Autodesk Inventor part; units mm, degrees
(part 2 of 2)
  spline S171 degree 2 poles (10.8818, -199.8751) (10.7521, -199.927) (10.5113, -200.0752) (10.4372, -200.1271) knots 0 0 0 1 2 2 2
  line L143 (10.4372, -200.1271) -> (10.4038, -200.1271)
  line L144 (10.4038, -200.1271) -> (10.4038, -199.475)
  spline S172 degree 2 poles (10.4038, -199.475) (10.5928, -199.3824) (11.2708, -199.2008) (11.5746, -199.2008) knots 0 0 0 1 2 2 2
  spline S173 degree 2 poles (11.5746, -199.2008) (12.2156, -199.2008) (12.938, -199.8788) (12.938, -200.4568) knots 0 0 0 1 2 2 2
  spline S174 degree 2 poles (12.938, -200.4568) (12.938, -200.7273) (12.8121, -201.1793) (12.7009, -201.372) knots 0 0 0 1 2 2 2
  spline S175 degree 2 poles (12.7009, -201.372) (12.5898, -201.572) (12.2674, -201.9648) (12.0896, -202.1537) knots 0 0 0 1 2 2 2
  spline S176 degree 2 poles (12.0896, -202.1537) (11.8006, -202.4686) (11.0929, -203.143) (10.8818, -203.3393) knots 0 0 0 1 2 2 2
  line L145 (10.8818, -203.3393) -> (13.127, -203.3393)
  line L146 (13.127, -203.3393) -> (13.127, -203.8691)
  line L147 (16.6801, -202.2982) -> (16.1355, -202.2982)
  line L148 (16.1355, -202.2982) -> (16.1355, -203.8691)
  line L149 (16.1355, -203.8691) -> (15.5464, -203.8691)
  line L150 (15.5464, -203.8691) -> (15.5464, -202.2982)
  line L151 (15.5464, -202.2982) -> (13.5271, -202.2982)
  line L152 (13.5271, -202.2982) -> (13.5271, -201.6535)
  line L153 (13.5271, -201.6535) -> (15.5723, -199.2971)
  line L154 (15.5723, -199.2971) -> (16.1355, -199.2971)
  line L155 (16.1355, -199.2971) -> (16.1355, -201.8054)
  line L156 (16.1355, -201.8054) -> (16.6801, -201.8054)
  line L157 (16.6801, -201.8054) -> (16.6801, -202.2982)
  line L158 (15.5464, -201.8054) -> (15.5464, -200.0196)
  line L159 (15.5464, -200.0196) -> (14.0088, -201.8054)
  line L160 (14.0088, -201.8054) -> (15.5464, -201.8054)
  line L161 (19.0699, -199.0934) -> (17.2803, -204.8621)
  line L162 (17.2803, -204.8621) -> (16.7616, -204.8621)
  line L163 (16.7616, -204.8621) -> (18.5437, -199.0934)
  line L164 (18.5437, -199.0934) -> (19.0699, -199.0934)
  line L165 (22.3933, -203.8691) -> (19.5737, -203.8691)
  line L166 (19.5737, -203.8691) -> (19.5737, -203.2208)
  spline S177 degree 2 poles (19.5737, -203.2208) (19.8776, -202.9355) (20.4185, -202.4057) (20.6778, -202.1204) knots 0 0 0 1 2 2 2
  spline S178 degree 2 poles (20.6778, -202.1204) (21.2003, -201.5461) (21.5819, -200.857) (21.5819, -200.4902) knots 0 0 0 1 2 2 2
  spline S179 degree 2 poles (21.5819, -200.4902) (21.5819, -200.2975) (21.4633, -200.0085) (21.3559, -199.9159) knots 0 0 0 1 2 2 2
  spline S180 degree 2 poles (21.3559, -199.9159) (21.2484, -199.8233) (20.9668, -199.7306) (20.7964, -199.7306) knots 0 0 0 1 2 2 2
  spline S181 degree 2 poles (20.7964, -199.7306) (20.6334, -199.7306) (20.2999, -199.8121) (20.148, -199.8751) knots 0 0 0 1 2 2 2
  spline S182 degree 2 poles (20.148, -199.8751) (20.0183, -199.927) (19.7775, -200.0752) (19.7034, -200.1271) knots 0 0 0 1 2 2 2
  line L167 (19.7034, -200.1271) -> (19.6701, -200.1271)
  line L168 (19.6701, -200.1271) -> (19.6701, -199.475)
  spline S183 degree 2 poles (19.6701, -199.475) (19.859, -199.3824) (20.5371, -199.2008) (20.8409, -199.2008) knots 0 0 0 1 2 2 2
  spline S184 degree 2 poles (20.8409, -199.2008) (21.4818, -199.2008) (22.2043, -199.8788) (22.2043, -200.4568) knots 0 0 0 1 2 2 2
  spline S185 degree 2 poles (22.2043, -200.4568) (22.2043, -200.7273) (22.0783, -201.1793) (21.9672, -201.372) knots 0 0 0 1 2 2 2
  spline S186 degree 2 poles (21.9672, -201.372) (21.856, -201.572) (21.5337, -201.9648) (21.3559, -202.1537) knots 0 0 0 1 2 2 2
  spline S187 degree 2 poles (21.3559, -202.1537) (21.0669, -202.4686) (20.3592, -203.143) (20.148, -203.3393) knots 0 0 0 1 2 2 2
  line L169 (20.148, -203.3393) -> (22.3933, -203.3393)
  line L170 (22.3933, -203.3393) -> (22.3933, -203.8691)
  spline S188 degree 2 poles (25.8501, -201.5831) (25.8501, -202.8132) (25.135, -203.9655) (24.3903, -203.9655) knots 0 0 0 1 2 2 2
  spline S189 degree 2 poles (24.3903, -203.9655) (23.6345, -203.9655) (22.9268, -202.791) (22.9268, -201.5868) knots 0 0 0 1 2 2 2
  spline S190 degree 2 poles (22.9268, -201.5868) (22.9268, -200.3494) (23.6419, -199.2045) (24.3903, -199.2045) knots 0 0 0 1 2 2 2
  spline S191 degree 2 poles (24.3903, -199.2045) (25.1424, -199.2045) (25.8501, -200.3901) (25.8501, -201.5831) knots 0 0 0 1 2 2 2
  spline S192 degree 2 poles (25.0646, -202.9762) (25.1535, -202.7502) (25.2276, -202.0537) (25.2276, -201.5831) knots 0 0 0 1 2 2 2
  spline S193 degree 2 poles (25.2276, -201.5831) (25.2276, -201.1126) (25.1535, -200.4198) (25.0609, -200.1863) knots 0 0 0 1 2 2 2
  spline S194 degree 2 poles (25.0609, -200.1863) (24.9683, -199.9529) (24.6459, -199.7121) (24.3903, -199.7121) knots 0 0 0 1 2 2 2
  spline S195 degree 2 poles (24.3903, -199.7121) (24.1346, -199.7121) (23.8049, -199.9529) (23.7086, -200.1938) knots 0 0 0 1 2 2 2
  spline S196 degree 2 poles (23.7086, -200.1938) (23.6159, -200.4272) (23.5492, -201.1385) (23.5492, -201.5868) knots 0 0 0 1 2 2 2
  spline S197 degree 2 poles (23.5492, -201.5868) (23.5492, -202.0685) (23.6085, -202.7132) (23.7048, -202.9651) knots 0 0 0 1 2 2 2
  spline S198 degree 2 poles (23.7048, -202.9651) (23.7938, -203.2022) (24.1235, -203.4579) (24.3903, -203.4579) knots 0 0 0 1 2 2 2
  spline S199 degree 2 poles (24.3903, -203.4579) (24.6422, -203.4579) (24.972, -203.2171) (25.0646, -202.9762) knots 0 0 0 1 2 2 2
  line L171 (29.255, -203.8691) -> (26.4355, -203.8691)
  line L172 (26.4355, -203.8691) -> (26.4355, -203.2208)
  spline S200 degree 2 poles (26.4355, -203.2208) (26.7393, -202.9355) (27.2802, -202.4057) (27.5395, -202.1204) knots 0 0 0 1 2 2 2
  spline S201 degree 2 poles (27.5395, -202.1204) (28.062, -201.5461) (28.4436, -200.857) (28.4436, -200.4902) knots 0 0 0 1 2 2 2
  spline S202 degree 2 poles (28.4436, -200.4902) (28.4436, -200.2975) (28.325, -200.0085) (28.2176, -199.9159) knots 0 0 0 1 2 2 2
  spline S203 degree 2 poles (28.2176, -199.9159) (28.1101, -199.8233) (27.8285, -199.7306) (27.6581, -199.7306) knots 0 0 0 1 2 2 2
  spline S204 degree 2 poles (27.6581, -199.7306) (27.4951, -199.7306) (27.1616, -199.8121) (27.0097, -199.8751) knots 0 0 0 1 2 2 2
  spline S205 degree 2 poles (27.0097, -199.8751) (26.8801, -199.927) (26.6392, -200.0752) (26.5651, -200.1271) knots 0 0 0 1 2 2 2
  line L173 (26.5651, -200.1271) -> (26.5318, -200.1271)
  line L174 (26.5318, -200.1271) -> (26.5318, -199.475)
  spline S206 degree 2 poles (26.5318, -199.475) (26.7207, -199.3824) (27.3988, -199.2008) (27.7026, -199.2008) knots 0 0 0 1 2 2 2
  spline S207 degree 2 poles (27.7026, -199.2008) (28.3435, -199.2008) (29.066, -199.8788) (29.066, -200.4568) knots 0 0 0 1 2 2 2
  spline S208 degree 2 poles (29.066, -200.4568) (29.066, -200.7273) (28.94, -201.1793) (28.8289, -201.372) knots 0 0 0 1 2 2 2
  spline S209 degree 2 poles (28.8289, -201.372) (28.7177, -201.572) (28.3954, -201.9648) (28.2176, -202.1537) knots 0 0 0 1 2 2 2
  spline S210 degree 2 poles (28.2176, -202.1537) (27.9286, -202.4686) (27.2209, -203.143) (27.0097, -203.3393) knots 0 0 0 1 2 2 2
  line L175 (27.0097, -203.3393) -> (29.255, -203.3393)
  line L176 (29.255, -203.3393) -> (29.255, -203.8691)
  spline S211 degree 2 poles (32.7562, -202.3871) (32.7562, -202.7391) (32.5228, -203.3356) (32.3264, -203.5357) knots 0 0 0 1 2 2 2
  spline S212 degree 2 poles (32.3264, -203.5357) (32.1227, -203.7469) (31.6114, -203.9655) (31.3039, -203.9655) knots 0 0 0 1 2 2 2
  spline S213 degree 2 poles (31.3039, -203.9655) (30.9963, -203.9655) (30.4887, -203.758) (30.2961, -203.5505) knots 0 0 0 1 2 2 2
  spline S214 degree 2 poles (30.2961, -203.5505) (30.059, -203.3023) (29.7922, -202.4686) (29.7922, -201.861) knots 0 0 0 1 2 2 2
  spline S215 degree 2 poles (29.7922, -201.861) (29.7922, -201.2645) (30.0367, -200.3049) (30.2924, -199.9492) knots 0 0 0 1 2 2 2
  spline S216 degree 2 poles (30.2924, -199.9492) (30.5406, -199.601) (31.3261, -199.2119) (31.8411, -199.2119) knots 0 0 0 1 2 2 2
  spline S217 degree 2 poles (31.8411, -199.2119) (31.993, -199.2119) (32.2597, -199.2416) (32.3598, -199.2749) knots 0 0 0 1 2 2 2
  line L177 (32.3598, -199.2749) -> (32.3598, -199.864)
  line L178 (32.3598, -199.864) -> (32.3338, -199.864)
  spline S218 degree 2 poles (32.3338, -199.864) (32.2486, -199.8196) (31.9374, -199.7417) (31.7596, -199.7417) knots 0 0 0 1 2 2 2
  spline S219 degree 2 poles (31.7596, -199.7417) (31.189, -199.7417) (30.4887, -200.5124) (30.4221, -201.2682) knots 0 0 0 1 2 2 2
  spline S220 degree 2 poles (30.4221, -201.2682) (30.6407, -201.1163) (31.1001, -200.9496) (31.3742, -200.9496) knots 0 0 0 1 2 2 2
  spline S221 degree 2 poles (31.3742, -200.9496) (31.641, -200.9496) (32.0412, -201.057) (32.2597, -201.22) knots 0 0 0 1 2 2 2
  spline S222 degree 2 poles (32.2597, -201.22) (32.5117, -201.409) (32.7562, -201.9944) (32.7562, -202.3871) knots 0 0 0 1 2 2 2
  spline S223 degree 2 poles (32.1338, -202.4131) (32.1338, -202.1315) (31.9856, -201.7499) (31.8226, -201.6165) knots 0 0 0 1 2 2 2
  spline S224 degree 2 poles (31.8226, -201.6165) (31.7003, -201.5202) (31.3965, -201.4572) (31.2372, -201.4572) knots 0 0 0 1 2 2 2
  spline S225 degree 2 poles (31.2372, -201.4572) (31.0223, -201.4572) (30.6184, -201.5868) (30.4221, -201.7091) knots 0 0 0 1 2 2 2
  spline S226 degree 2 poles (30.4221, -201.7091) (30.4184, -201.7758) (30.4109, -201.9018) (30.4109, -201.9981) knots 0 0 0 1 2 2 2
  spline S227 degree 2 poles (30.4109, -201.9981) (30.4109, -202.4723) (30.5962, -203.054) (30.737, -203.2059) knots 0 0 0 1 2 2 2
  spline S228 degree 2 poles (30.737, -203.2059) (30.8667, -203.3504) (31.1482, -203.4653) (31.3076, -203.4653) knots 0 0 0 1 2 2 2
  spline S229 degree 2 poles (31.3076, -203.4653) (31.6781, -203.4653) (32.1338, -202.9392) (32.1338, -202.4131) knots 0 0 0 1 2 2 2
  point P0 (0, 0)
  constraints: 2 other
emboss "Emboss1" sketch "Sketch14" operation cut depth 2.54 direction (-1, 0, 0)
sketch "Sketch16" plane through (5.08, 0, 0) normal (1, 0, 0) x (0, 0, -1)
  line L0 (-45.5467, -73.9362) -> (38.2733, -73.9362)
  line L1 (38.2733, -73.9362) -> (38.2733, -77.7462)
  line L2 (38.2733, -77.7462) -> (-45.5467, -77.7462)
  line L3 (-45.5467, -77.7462) -> (-45.5467, -73.9362)
  line L4 (38.9083, -211.0962) -> (-46.1817, -211.0962) projected
  line L5 (42.0833, 28.0448) -> (42.0833, -207.9212) projected
  line L6 (-49.3567, -207.9212) -> (-49.3567, 28.0448) projected
  point P0 (0, 0)
  point P1 (38.9083, -223.7962)
  point P2 (42.0833, -220.6212)
  point P3 (38.2733, -75.8412)
  point P4 (-45.5467, -75.8412)
  dimension "d195" = 3.81
  dimension "d692" = 137.16
  dimension "d796" = 3.81
  dimension "d797" = 3.81
  constraints: 8 end point, 2 midpoint, 2 parallel, 1 horizontal, 1 perpendicular, 1 other
  measures "d195" distance between parallel lines of L0 L2
  measures "d796" distance from line of L5 point (38.273, -75.841)
  measures "d797" distance from line of L6 point (-45.547, -75.841)
extrude "Extrusion13" add sketch "Sketch16" along normal blind 5.08
sketch "Sketch17" plane through (24.13, 33.2264, 43.0067) normal (0, 1, 0) x (1, 0, 0)
  line L0 (-8.128, 57.15) -> (0, 57.15) projected
  line L1 (-0.0061, 57.15) -> (0.0392, 57.15)
  line L2 (0, 87.0966) -> (0, -8.3566) projected
  line L3 (0, 35.5801) -> (0, 35.5243)
  line L4 (5, -5.1816) -> (5, 83.9216) projected
  line L5 (0, 57.15) -> (5, 57.15)
  line L6 (5, 57.15) -> (5, 0)
  line L7 (5, 0) -> (0, 0)
  line L8 (0, 0) -> (0, 57.15)
  line L9 (0, 0) -> (-8.128, 0) projected
  point P0 (-24.13, 43.0067)
  point P1 (5, -23.8506)
  point P2 (5, 69.0626)
  point P3 (0, 0)
  point P4 (5, 57.15)
  point P5 (2.5, 0)
  point P6 (2.5, 57.15)
  dimension "d689" = 57.15
  dimension "d1196" = 0
  constraints: 12 end point, 4 point on line, 2 horizontal, 2 midpoint, 2 parallel, 1 perpendicular
  measures "d689" distance of point (2.5, 0) point (2.5, 57.15)
  measures "d1196" distance between parallel lines of L7 L9
extrude "Extrusion14" cut sketch "Sketch17" against normal blind 2.0066
sketch "Sketch18" plane through (0, 0, 0) normal (-1, 0, 0) x (0, 0, 1)
  arc A0 (48.3408, 33.2227) -> (51.3596, 30.2039) centre (50.6267, 32.4898) ccw projected
  circle A1 centre (50.6267, 32.4898) radius 4.5085
  arc A2 (-41.0674, 33.2227) -> (-44.0862, 30.2039) centre (-43.3533, 32.4898) ccw projected
  circle A3 centre (-43.3533, 32.4898) radius 4.5085
  arc A4 (-44.0862, -210.0804) -> (-41.0674, -213.0992) centre (-43.3533, -212.3662) ccw projected
  circle A5 centre (-43.3533, -212.3662) radius 4.5085
  arc A6 (48.3408, -213.0992) -> (51.3596, -210.0804) centre (50.6267, -212.3662) ccw projected
  circle A7 centre (50.6267, -212.3662) radius 4.5085
  point P0 (0, 0)
  point P1 (-44.0899, -199.9215)
  point P2 (-44.0899, -204.4909)
  point P3 (51.3633, -204.4909)
  point P4 (51.3633, -199.9215)
  point P5 (-41.0686, 33.2264)
  point P6 (-41.0686, -213.1028)
  dimension "d209" = 9.017
  dimension "d210" = 9.017
  dimension "d211" = 9.017
  dimension "d212" = 9.017
  constraints: 4 centre point, 4 coincident
  measures "d209" diameter of A1
  measures "d210" diameter of A3
  measures "d211" diameter of A5
  measures "d212" diameter of A7
extrude "Extrusion15" [suppressed]
sketch "Sketch19" plane through (24.13, -51.5842, -44.0899) normal (0, 0, -1) x (-1, 0, 0)
  line L0 (7.62, 0) -> (0, 0) projected
  line L1 (-5, 79.629) -> (-5, -156.337) projected
  line L2 (0, 0) -> (-5, 0)
  line L3 (-5, 0) -> (-5, 12.7)
  line L4 (-5, 12.7) -> (0, 12.7)
  line L5 (0, 12.7) -> (0, 0)
  point P0 (24.13, 51.5842)
  point P1 (-5, -156.337)
  dimension "d216" = 5
  dimension "d219" = 12.7
  constraints: 8 end point, 2 parallel, 1 horizontal, 1 perpendicular, 1 point on line
  measures "d216" distance between parallel lines of L1 L5
  measures "d219" distance between parallel lines of L2 L4
extrude "Extrusion16" cut sketch "Sketch19" against normal blind 24.13
sketch "Sketch20" plane through (0, 0, 0) normal (-1, 0, 0) x (0, 0, 1)
  line L0 (-45.1249, 28.9592) -> (-41.5943, 28.9592)
  line L1 (-45.1249, 36.0204) -> (-41.5943, 36.0204)
  line L2 (-45.1249, 28.9592) -> (-47.1633, 32.4898)
  line L3 (-45.1249, 36.0204) -> (-47.1633, 32.4898)
  line L4 (-41.5943, 28.9592) -> (-39.5559, 32.4898)
  line L5 (-41.5943, 36.0204) -> (-39.5559, 32.4898)
  line L6 (48.8551, 28.9592) -> (52.3857, 28.9592)
  line L7 (48.8551, 36.0204) -> (52.3857, 36.0204)
  line L8 (48.8551, 28.9592) -> (46.8167, 32.4898)
  line L9 (48.8551, 36.0204) -> (46.8167, 32.4898)
  line L10 (52.3857, 28.9592) -> (54.4241, 32.4898)
  line L11 (52.3857, 36.0204) -> (54.4241, 32.4898)
  line L12 (-40.6799, -67.5608) -> (-37.1493, -67.5608)
  line L13 (-40.6799, -60.4996) -> (-37.1493, -60.4996)
  line L14 (-40.6799, -67.5608) -> (-42.7183, -64.0302)
  line L15 (-40.6799, -60.4996) -> (-42.7183, -64.0302)
  line L16 (-37.1493, -67.5608) -> (-35.1109, -64.0302)
  line L17 (-37.1493, -60.4996) -> (-35.1109, -64.0302)
  line L18 (44.4101, -67.5608) -> (47.9407, -67.5608)
  line L19 (44.4101, -60.4996) -> (47.9407, -60.4996)
  line L20 (44.4101, -67.5608) -> (42.3717, -64.0302)
  line L21 (44.4101, -60.4996) -> (42.3717, -64.0302)
  line L22 (47.9407, -67.5608) -> (49.9791, -64.0302)
  line L23 (47.9407, -60.4996) -> (49.9791, -64.0302)
  line L24 (48.8551, -215.8968) -> (52.3857, -215.8968)
  line L25 (48.8551, -208.8356) -> (52.3857, -208.8356)
  line L26 (48.8551, -215.8968) -> (46.8167, -212.3662)
  line L27 (48.8551, -208.8356) -> (46.8167, -212.3662)
  line L28 (52.3857, -215.8968) -> (54.4241, -212.3662)
  line L29 (52.3857, -208.8356) -> (54.4241, -212.3662)
  line L30 (-45.1249, -215.8968) -> (-41.5943, -215.8968)
  line L31 (-45.1249, -208.8356) -> (-41.5943, -208.8356)
  line L32 (-45.1249, -215.8968) -> (-47.1633, -212.3662)
  line L33 (-45.1249, -208.8356) -> (-47.1633, -212.3662)
  line L34 (-41.5943, -215.8968) -> (-39.5559, -212.3662)
  line L35 (-41.5943, -208.8356) -> (-39.5559, -212.3662)
  point P0 (0, 0)
  point P1 (-16.6833, 31.2198)
  point P2 (-43.3596, 28.9592)
  point P3 (-43.3533, 32.4898)
  point P4 (50.6204, 28.9592)
  point P5 (-38.9146, -67.5608)
  point P6 (-38.9083, -64.0302)
  point P7 (46.1754, -67.5608)
  point P8 (46.1817, -64.0302)
  point P9 (50.6204, -215.8968)
  point P10 (-43.3596, -215.8968)
  dimension "d963" = 7.0612
  dimension "d964" = 120
  dimension "d965" = 120
  dimension "d966" = 120
  dimension "d967" = 120
  dimension "d968" = 3.5306
  dimension "d969" = 3.5306
  dimension "d970" = 3.5306
  dimension "d971" = 3.5306
  dimension "d972" = 3.5306
  dimension "d973" = 3.5306
  dimension "d974" = 0
  dimension "d975" = 7.6074
  dimension "d1082" = 7.0612
  dimension "d1083" = 120
  dimension "d1084" = 120
  dimension "d1085" = 120
  dimension "d1086" = 120
  dimension "d1087" = 3.5306
  dimension "d1088" = 3.5306
  dimension "d1089" = 3.5306
  dimension "d1090" = 3.5306
  dimension "d1091" = 3.5306
  dimension "d1092" = 3.5306
  dimension "d1093" = 0
  dimension "d1094" = 7.6074
  dimension "d1301" = 7.0612
  dimension "d1302" = 120
  dimension "d1303" = 120
  dimension "d1304" = 120
  dimension "d1305" = 120
  dimension "d1306" = 3.5306
  dimension "d1307" = 3.5306
  dimension "d1308" = 3.5306
  dimension "d1309" = 3.5306
  dimension "d1310" = 3.5306
  dimension "d1311" = 3.5306
  dimension "d1312" = 0
  dimension "d1313" = 7.6074
  dimension "d1318" = 7.0612
  dimension "d1319" = 120
  dimension "d1320" = 120
  dimension "d1321" = 120
  dimension "d1322" = 120
  dimension "d1323" = 3.5306
  dimension "d1324" = 3.5306
  dimension "d1325" = 3.5306
  dimension "d1326" = 3.5306
  dimension "d1327" = 3.5306
  dimension "d1328" = 3.5306
  dimension "d1329" = 0
  dimension "d1330" = 7.6074
  dimension "d1335" = 7.0612
  dimension "d1336" = 120
  dimension "d1337" = 120
  dimension "d1338" = 120
  dimension "d1339" = 120
  dimension "d1340" = 3.5306
  dimension "d1341" = 3.5306
  dimension "d1342" = 3.5306
  dimension "d1343" = 3.5306
  dimension "d1344" = 3.5306
  dimension "d1345" = 3.5306
  dimension "d1346" = 0
  constraints: 72 end point, 12 horizontal, 6 midpoint
  measures "d963" distance from line of point (-43.36, 28.959) L1
  measures "d964" angle of L0 L2
  measures "d965" angle of L1 L3
  measures "d966" angle of L4 L0
  measures "d967" angle of L5 L1
  measures "d968" distance of L0.start L4.start
  measures "d969" distance of L1.start L5.start
  measures "d970" vertical distance of L1.start L3.end
  measures "d971" vertical distance of L0.start L2.end
  measures "d972" vertical distance of L5.start L5.end
  measures "d973" vertical distance of L4.start L4.end
  measures "d974" horizontal distance of L0.start L1.start
  measures "d975" distance of L4.end L2.end
  measures "d1082" distance from line of point (50.62, 28.959) L7
  measures "d1083" angle of L6 L8
  measures "d1084" angle of L7 L9
  measures "d1085" angle of L10 L6
  measures "d1086" angle of L11 L7
  measures "d1087" distance of L6.start L10.start
  measures "d1088" distance of L9.start L11.start
  measures "d1089" vertical distance of L9.start L9.end
  measures "d1090" vertical distance of L6.start L8.end
  measures "d1091" vertical distance of L11.start L11.end
  measures "d1092" vertical distance of L10.start L10.end
  measures "d1093" horizontal distance of L6.start L9.start
  measures "d1094" distance of L10.end L8.end
  measures "d1301" distance from line of point (-38.915, -67.561) L13
  measures "d1302" angle of L12 L14
  measures "d1303" angle of L13 L15
  measures "d1304" angle of L16 L12
  measures "d1305" angle of L17 L13
  measures "d1306" distance of L12.start L16.start
  measures "d1307" distance of L13.start L17.start
  measures "d1308" vertical distance of L13.start L15.end
  measures "d1309" vertical distance of L12.start L14.end
  measures "d1310" vertical distance of L17.start L17.end
  measures "d1311" vertical distance of L16.start L16.end
  measures "d1312" horizontal distance of L12.start L13.start
  measures "d1313" distance of L16.end L14.end
  measures "d1318" distance from line of point (46.175, -67.561) L19
  measures "d1319" angle of L18 L20
  measures "d1320" angle of L19 L21
  measures "d1321" angle of L22 L18
  measures "d1322" angle of L23 L19
  measures "d1323" distance of L18.start L22.start
  measures "d1324" distance of L19.start L23.start
  measures "d1325" vertical distance of L19.start L21.end
  measures "d1326" vertical distance of L18.start L20.end
  measures "d1327" vertical distance of L23.start L23.end
  measures "d1328" vertical distance of L22.start L22.end
  measures "d1329" horizontal distance of L18.start L19.start
  measures "d1330" distance of L22.end L20.end
  measures "d1335" distance from line of point (50.62, -215.897) L25
  measures "d1336" angle of L24 L26
  measures "d1337" angle of L25 L27
  measures "d1338" angle of L28 L24
  measures "d1339" angle of L29 L25
  measures "d1340" distance of L24.start L28.start
  measures "d1341" distance of L25.start L29.start
  measures "d1342" vertical distance of L25.start L27.end
  measures "d1343" vertical distance of L24.start L26.end
  measures "d1344" vertical distance of L29.start L29.end
  measures "d1345" vertical distance of L28.start L28.end
  measures "d1346" horizontal distance of L24.start L25.start
extrude "Extrusion18" cut sketch "Sketch20" against normal blind 4
sketch "Sketch21" plane through (5.08, 0, 0) normal (1, 0, 0) x (0, 0, -1)
  line L0 (-49.3567, -207.9212) -> (-49.3567, 28.0448) projected
  line L1 (42.0833, -69.6717) -> (42.0833, -83.8957)
  line L2 (44.0899, -209.9278) -> (44.0899, -51.5842) projected
  line L3 (-49.3567, -83.8422) -> (-49.3567, -69.6182)
  line L4 (-42.4987, -58.8939) -> (-42.4987, -69.23)
  line L5 (-44.2301, -72.0578) -> (-47.3797, -73.6657)
  line L6 (-48.7308, -74.9867) -> (-49.3567, -76.1476)
  line L7 (-44.2301, -56.0661) -> (-47.3797, -54.4582)
  line L8 (-48.7639, -53.074) -> (-49.3567, -51.9128)
  arc A0 (-47.3797, -73.6657) -> (-48.7308, -74.9867) centre (-45.9361, -76.4935) ccw
  arc A1 (-44.2301, -72.0578) -> (-42.4987, -69.23) centre (-45.6737, -69.23) ccw
  arc A2 (-42.4987, -58.8939) -> (-44.2301, -56.0661) centre (-45.6737, -58.8939) ccw
  arc A3 (-48.7639, -53.074) -> (-47.3797, -54.4582) centre (-45.9361, -51.6304) ccw
  line L9 (-49.3567, -51.9128) -> (-49.3567, -76.1476)
  line L10 (35.2253, -69.1835) -> (35.2253, -58.8478)
  line L11 (36.9569, -56.0198) -> (40.1065, -54.4123)
  line L12 (41.4675, -53.0729) -> (42.0833, -51.9128)
  line L13 (36.9569, -72.0115) -> (40.1065, -73.619)
  line L14 (41.4675, -74.9584) -> (42.0833, -76.1184)
  arc A4 (41.4675, -74.9584) -> (40.1065, -73.619) centre (38.6631, -76.447) ccw
  arc A5 (35.2253, -69.1835) -> (36.9569, -72.0115) centre (38.4003, -69.1835) ccw
  arc A6 (40.1065, -54.4123) -> (41.4675, -53.0729) centre (38.6631, -51.5843) ccw
  arc A7 (36.9569, -56.0198) -> (35.2253, -58.8478) centre (38.4003, -58.8478) ccw
  line L15 (42.0833, -51.9128) -> (42.0833, -76.1184)
  line L16 (42.0833, -51.9128) -> (42.0833, -76.1184)
  circle A8 centre (38.9083, -64.0302) radius 2.4005 projected
  line L17 (42.0833, -51.5842) -> (42.0833, -38.8842) projected
  circle A9 centre (38.9083, -64.0302) radius 2.4005
  circle A10 centre (-46.1817, -64.0302) radius 2.4005 projected
  circle A11 centre (-46.1817, -64.0302) radius 2.4005
  point P0 (0, 0)
  point P1 (-43.0067, -58.9502)
  point P2 (-48.2611, -74.1156)
  point P3 (-48.2961, -53.9904)
  point P4 (-43.0067, -74.3297)
  point P5 (-40.8318, -77.7462)
  point P6 (-48.5822, -64.0302)
  point P7 (-48.5822, -64.0302)
  point P8 (-48.5822, -64.0302)
  point P9 (-48.5822, -64.0302)
  point P10 (40.9982, -53.9572)
  point P11 (42.0833, -76.1184)
  point P12 (35.8863, -63.7762)
  point P13 (38.2733, -66.4307)
  dimension "d785" = 6.858
  dimension "d786" = 117.044
  dimension "d787" = 117.044
  dimension "d792" = 2.032
  dimension "d793" = 3.175
  dimension "d794" = 3.1496
  dimension "d795" = 3.1496
  dimension "d917" = 24.2348
  dimension "d1144" = 145
  dimension "d1145" = 145
  dimension "d1146" = 117.04
  dimension "d1147" = 117.04
  dimension "d1148" = 3.175
  dimension "d1149" = 3.175
  dimension "d1150" = 3.1496
  dimension "d1151" = 2.0443
  dimension "d1152" = 3.1496
  dimension "d1153" = 24.2056
  dimension "d1155" = 0
  dimension "d1159" = 12.1174
  dimension "d1198" = 12.1174
  constraints: 30 end point, 16 point on circle, 16 tangent, 10 centre point, 9 point on line, 5 equal radius, 2 coincident, 2 vertical, 1 collinear, 1 concentric, 1 parallel, 1 perpendicular, 2 other
  measures "d785" distance between parallel lines of L0 L4
  measures "d786" angle of L5 L4
  measures "d787" angle of L7 L4
  measures "d792" vertical distance of point (-48.261, -74.116) L6.end
  measures "d793" radius of A0
  measures "d794" horizontal distance of L5.start L5.end
  measures "d795" horizontal distance of L7.start L7.end
  measures "d917" distance of L6.end L8.end
  measures "d1144" angle of L11 L12
  measures "d1145" angle of L14 L13
  measures "d1146" angle of L13 L10
  measures "d1147" angle of L10 L11
  measures "d1148" radius of A4
  measures "d1149" radius of A6
  measures "d1150" horizontal distance of L11.start L11.end
  measures "d1151" vertical distance of L12.end point (40.998, -53.957)
  measures "d1152" horizontal distance of L13.start L13.end
  measures "d1153" distance of L14.end L12.end
  measures "d1155" distance between parallel lines of L17 L15
  measures "d1159" vertical distance of point (38.908, -64.03) L12.end
  measures "d1198" vertical distance of A10.centre L8.end
extrude "Extrusion19" add sketch "Sketch21" along normal blind 24.13
sketch "Sketch22" plane through (16.08, -230.1462, -3.2973) normal (0, -1, 0) x (1, 0, 0)
  circle A0 centre (2.2292, -12.1283) radius 2.032
  line L0 (-16.08, -45.136) -> (8.05, -45.136) projected
  circle A1 centre (10.002, -12.1283) radius 2.032
  line L1 (13.05, 48.9456) -> (13.05, -37.6176) projected
  point P0 (-16.08, 3.2973)
  dimension "d445" = 4.064
  dimension "d446" = 33.0076
  dimension "d449" = 4.064
  dimension "d450" = 3.048
  constraints: 2 centre point
  measures "d445" diameter of A0
  measures "d446" distance from line of L0 A0.centre
  measures "d449" diameter of A1
  measures "d450" distance from line of L1 A1.centre
extrude "Extrusion20" [suppressed]
fillet "Fillet6" radius 0.508 5 edges at (20.32, -51.5842, -48.4333) (16.51, -45.2342, -48.4333) (20.32, -38.8842, -48.4333) (20.066, 37.5698, -14.1433) (16.002, 37.5698, 14.4317)
sketch "Sketch23" plane through (22.86, -225.8028, -3.2973) normal (0, -1, 0) x (1, 0, 0)
  line L0 (1.27, -37.6176) -> (1.27, 48.9456) projected
  line L1 (6.27, 48.9456) -> (6.27, -37.6176) projected
  line L2 (0, 10) -> (6.27, 10)
  line L3 (6.27, 10) -> (6.27, -0.0129)
  line L4 (6.27, -0.0129) -> (0, -0.0129)
  line L5 (0, -0.0129) -> (0, 10)
  point P0 (-22.86, 3.2973)
  point P1 (1.27, 48.9456)
  constraints: 8 end point, 2 parallel, 1 horizontal, 1 perpendicular, 1 point on line, 1 other
extrude "Extrusion21" [suppressed]
sketch "Sketch24" plane through (8.636, -223.7962, -3.2973) normal (0, 1, 0) x (1, 0, 0)
  circle A0 centre (9.652, -31.318) radius 4.445
  line L0 (-3.556, 35.611) -> (-3.556, -46.939) projected
  point P0 (-8.636, -3.2973)
  point P1 (15.494, -56.464)
  dimension "d673" = 25.146
  dimension "d674" = 13.208
  dimension "d677" = 8.89
  constraints: 1 centre point
  measures "d673" vertical distance of point (15.494, -56.464) A0.centre
  measures "d674" distance from line of L0 A0.centre
  measures "d677" diameter of A0
extrude "Extrusion22" [suppressed]
sketch "Sketch25" plane through (5.08, 0, 0) normal (1, 0, 0) x (0, 0, -1)
  line L0 (-49.3567, 15.9798) -> (20.6609, 15.9798)
  line L1 (11.7709, 3.2798) -> (-49.3567, 3.2798)
  line L2 (-49.3567, 3.2798) -> (-49.3567, 15.9798)
  circle A0 centre (-32.8467, 9.6298) radius 2.4005 projected
  circle A1 centre (4.1509, 9.6298) radius 2.4005 projected
  circle A2 centre (-14.3479, 9.6298) radius 2.4005 projected
  line L3 (-49.3567, -207.9212) -> (-49.3567, 28.0448) projected
  line L4 (42.0833, 28.0448) -> (42.0833, -38.8842) projected
  line L5 (20.6609, 15.9798) -> (42.0833, 15.9798)
  line L6 (42.0833, 15.9798) -> (42.0833, 3.2798)
  line L7 (42.0833, 3.2798) -> (11.7709, 3.2798)
  point P0 (0, 0)
  point P1 (-14.3479, 15.9798)
  point P2 (-46.8167, -36.8286)
  point P3 (-49.3567, 28.0448)
  point P4 (42.0833, -36.6918)
  point P5 (-49.3567, -207.9212)
  dimension "d680" = 6.35
  dimension "d681" = 6.35
  dimension "d682" = 0
  dimension "d685" = 0
  dimension "d686" = 12.7
  constraints: 12 end point, 2 horizontal, 2 parallel, 1 midpoint, 1 perpendicular, 1 other
  measures "d680" distance of point (-14.348, 15.98) A2.centre
  measures "d681" distance from line of L1 A2.centre
  measures "d682" horizontal extent of L2
  measures "d685" distance between parallel lines of L4 L6
  measures "d686" distance between parallel lines of L7 L5
extrude "Extrusion23" add sketch "Sketch25" along normal blind 10.16
sketch "Sketch26" plane through (0, -217.4462, -45.2583) normal (0, -1, 0) x (1, 0, 0)
  line L0 (29.13, 88.265) -> (10.3097, 88.265)
  line L1 (10.3097, 9.525) -> (29.13, 9.525)
  line L2 (29.13, 9.525) -> (29.13, 88.265)
  line L3 (0, -3.175) -> (24.13, -3.175) projected
  line L4 (24.13, 100.965) -> (0, 100.965) projected
  line L5 (29.13, 93.4466) -> (29.13, 4.3434) projected
  line L6 (8.7811, 88.265) -> (8.7811, 85.0428)
  line L7 (10.3097, 88.265) -> (8.7811, 88.265)
  line L8 (8.7811, 88.265) -> (8.7811, 9.525)
  line L9 (10.3097, 9.525) -> (8.7811, 9.525)
  point P0 (0, 45.2583)
  point P1 (29.13, 51.961)
  dimension "d832" = 12.7
  dimension "d833" = 12.7
  dimension "d837" = 0
  constraints: 14 end point, 2 horizontal, 2 perpendicular, 1 parallel, 1 vertical
  measures "d832" distance between parallel lines of L3 L1
  measures "d833" distance between parallel lines of L4 L0
  measures "d837" distance between parallel lines of L5 L2
extrude "Extrusion24" cut sketch "Sketch26" against normal blind 7.62
fillet "Fillet7" radius 0.762 4 edges at (17.2199, -217.4462, 43.0067) (9.5454, -217.4462, 43.0067) (17.2199, -217.4462, -35.7333) (9.5454, -217.4462, -35.7333)
body "Solid1"
